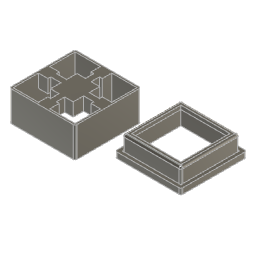
Eyebrow Warning Buttons v9 (Autodesk Fusion 360 design; units mm, degrees)
Autodesk Fusion 360 part; units mm, degrees
sketch "Sketch1" plane through (0, 0, 0) normal (0, 0, 1) x (1, 0, 0)
  line L0 (2.45, 3) -> (-2.45, 3)
  line L1 (-2.45, 3) -> (-2.45, -3)
  line L2 (-2.45, -3) -> (2.45, -3)
  line L3 (2.45, -3) -> (2.45, 3)
  line L4 (2.45, 3) -> (-2.45, -3) construction
  line L5 (-2.45, 3) -> (2.45, -3) construction
  line L6 (8.7, 8.7) -> (-8.7, 8.7)
  line L7 (-8.7, 8.7) -> (-8.7, -8.7)
  line L8 (-8.7, -8.7) -> (8.7, -8.7)
  line L9 (8.7, -8.7) -> (8.7, 8.7)
  line L10 (8.7, 8.7) -> (-8.7, -8.7) construction
  line L11 (-8.7, 8.7) -> (8.7, -8.7) construction
  line L12 (-8.7, 1.5) -> (-5.7, 1.5)
  line L13 (-5.7, 1.5) -> (-5.7, -1.5)
  line L14 (-5.7, -1.5) -> (-8.7, -1.5)
  line L15 (-8.7, -1.5) -> (-8.7, 1.5)
  line L16 (-1.5, 8.7) -> (1.5, 8.7)
  line L17 (1.5, 8.7) -> (1.5, 5.7)
  line L18 (1.5, 5.7) -> (-1.5, 5.7)
  line L19 (-1.5, 5.7) -> (-1.5, 8.7)
  line L20 (-1.5, -8.7) -> (1.5, -8.7)
  line L21 (1.5, -8.7) -> (1.5, -5.7)
  line L22 (1.5, -5.7) -> (-1.5, -5.7)
  line L23 (-1.5, -5.7) -> (-1.5, -8.7)
  line L24 (8.7, 1.5) -> (5.7, 1.5)
  line L25 (5.7, 1.5) -> (5.7, -1.5)
  line L26 (5.7, -1.5) -> (8.7, -1.5)
  line L27 (8.7, -1.5) -> (8.7, 1.5)
  line L28 (-8.2, 8.2) -> (8.2, 8.2)
  line L29 (8.2, 8.2) -> (8.2, -8.2)
  line L30 (8.2, -8.2) -> (-8.2, -8.2)
  line L31 (-8.2, -8.2) -> (-8.2, 8.2)
  line L32 (-8.2, 8.2) -> (8.2, -8.2) construction
  line L33 (8.2, 8.2) -> (-8.2, -8.2) construction
  line L34 (-3, 3.5) -> (3, 3.5)
  line L35 (3, 3.5) -> (3, -3.5)
  line L36 (3, -3.5) -> (-3, -3.5)
  line L37 (-3, -3.5) -> (-3, 3.5)
  line L38 (-3, 3.5) -> (3, -3.5) construction
  line L39 (3, 3.5) -> (-3, -3.5) construction
  line L40 (-6.05, 0.75) -> (-2.8, 0.75)
  line L41 (-2.8, 0.75) -> (-2.8, -0.75)
  line L42 (-2.8, -0.75) -> (-6.05, -0.75)
  line L43 (-6.05, -0.75) -> (-6.05, 0.75)
  line L44 (-0.75, -6.05) -> (0.75, -6.05)
  line L45 (0.75, -6.05) -> (0.75, -3.5)
  line L46 (0.75, -3.5) -> (-0.75, -3.5)
  line L47 (-0.75, -3.5) -> (-0.75, -6.05)
  line L48 (6.05, -0.75) -> (3, -0.75)
  line L49 (3, -0.75) -> (3, 0.75)
  line L50 (3, 0.75) -> (6.05, 0.75)
  line L51 (6.05, 0.75) -> (6.05, -0.75)
  line L52 (-0.75, 6.05) -> (0.75, 6.05)
  line L53 (0.75, 6.05) -> (0.75, 3.5)
  line L54 (0.75, 3.5) -> (-0.75, 3.5)
  line L55 (-0.75, 3.5) -> (-0.75, 6.05)
  point P0 (8.7, 0)
  point P1 (0, 8.7)
  point P2 (0, -8.7)
  point P3 (-5.7, 0)
  point P4 (0, -5.7)
  point P5 (5.7, 0)
  point P6 (0, 5.7)
  dimension "d1" = 4.9
  dimension "d2" = 6
  dimension "d3" = 17.4
  dimension "d4" = 17.4
  dimension "d7" = 3
  dimension "d8" = 3
  dimension "d15" = 3
  dimension "d16" = 3
  dimension "d17" = 3
  dimension "d18" = 3
  dimension "d19" = 3
  dimension "d20" = 3
  dimension "d21" = 16.4
  dimension "d22" = 16.4
  dimension "d23" = 6
  dimension "d24" = 7
  dimension "d31" = 1.5
  constraint horizontal L0
  constraint perpendicular L0 L1
  constraint parallel L0 L2
  constraint parallel L1 L3
  constraint coincident L4 origin
  constraint coincident L5 origin
  constraint horizontal L6
  constraint perpendicular L6 L7
  constraint parallel L6 L8
  constraint parallel L7 L9
  constraint coincident L10 origin
  constraint coincident L11 origin
  constraint horizontal L12
  constraint vertical L13
  constraint horizontal L14
  constraint vertical L15
  constraint midpoint L9 P0
  constraint midpoint L6 P1
  constraint midpoint L8 P2
  constraint horizontal L16
  constraint vertical L17
  constraint horizontal L18
  constraint vertical L19
  constraint horizontal L20
  constraint vertical L21
  constraint horizontal L22
  constraint vertical L23
  constraint horizontal L24
  constraint vertical L25
  constraint horizontal L26
  constraint vertical L27
  constraint horizontal L28
  constraint perpendicular L28 L29
  constraint parallel L28 L30
  constraint parallel L29 L31
  constraint coincident L32 origin
  constraint coincident L33 origin
  constraint horizontal L34
  constraint perpendicular L34 L35
  constraint parallel L34 L36
  constraint parallel L35 L37
  constraint coincident L38 origin
  constraint coincident L39 origin
  constraint midpoint L13 P3
  constraint horizontal L40
  constraint vertical L41
  constraint horizontal L42
  constraint vertical L43
  constraint midpoint L22 P4
  constraint horizontal L44
  constraint vertical L45
  constraint horizontal L46
  constraint vertical L47
  constraint coincident L36 L45.end
  constraint midpoint L25 P5
  constraint horizontal L48
  constraint vertical L49
  constraint horizontal L50
  constraint vertical L51
  constraint coincident L35 L49.end
  constraint midpoint L18 P6
  constraint horizontal L52
  constraint vertical L53
  constraint horizontal L54
  constraint vertical L55
  constraint coincident L34 L53.end
  measures "d1" distance of L1.end L2.end
  measures "d2" distance of L0.end L1.end
  measures "d3" distance of L7.end L8.end
  measures "d4" distance of L6.end L7.end
  measures "d7" distance of L12.start L12.end
  measures "d8" distance of L12.start L14.end
  measures "d15" distance of L16.start L16.end
  measures "d16" distance of L16.start L18.end
  measures "d17" distance of L20.start L20.end
  measures "d18" distance of L20.start L22.end
  measures "d19" distance of L24.start L24.end
  measures "d20" distance of L24.start L26.end
  measures "d21" distance of L29.end L30.end
  measures "d22" distance of L28.end L29.end
  measures "d23" distance of L35.end L36.end
  measures "d24" distance of L34.end L35.end
  measures "d31" distance of L40.start L42.end
extrude "Extrude1" add sketch "Sketch1" against normal blind 6.5 contours L6 L9 L17 L24 L28 L29 | L6 L16 L17 L19 L28 | L9 L24 L26 L27 L29 | L6 L7 L12 L19 L28 L31 | L17 L18 L19 L28 L52 L53 L55 | L8 L9 L21 L26 L29 L30 | L24 L25 L26 L29 L48 L50 L51 | L7 L12 L14 L15 L31 | L18 L52 L53 L55 | L8 L20 L21 L23 L30 | L25 L48 L50 L51 | L7 L8 L14 L23 L30 L31 | L12 L13 L14 L31 L40 L42 L43 | L21 L22 L23 L30 L44 L45 L47 | L13 L40 L42 L43 | L22 L44 L45 L47 makes body 1
fillet "Fillet1" radius 0.5 4 edges at (-8.7, 8.7, -3.25) (-8.7, -8.7, -3.25) (8.7, -8.7, -3.25) (8.7, 8.7, -3.25) on bodies 1
extrude "Extrude2" add sketch "Sketch1" against normal blind 2 separate body contours L18 L34 L53 L54 L55 | L25 L35 L48 L49 L50 | L34 L35 L36 L37 L40 L41 L42 L46 L49 L54 | L13 L37 L40 L42 | L22 L36 L45 L46 L47 | L37 L40 L41 L42 makes body 2
extrude "Extrude3" add sketch "Sketch1" along normal blind 1.5 contours L0 L1 L2 L3 | L6 L9 L17 L24 L28 L29 | L6 L16 L17 L19 L28 | L9 L24 L26 L27 L29 | L6 L7 L12 L19 L28 L31 | L17 L18 L19 L28 L52 L53 L55 | L8 L9 L21 L26 L29 L30 | L24 L25 L26 L29 L48 L50 L51 | L7 L12 L14 L15 L31 | L18 L34 L53 L54 L55 | L18 L52 L53 L55 | L8 L20 L21 L23 L30 | L25 L48 L50 L51 | L25 L35 L48 L49 L50 | L7 L8 L14 L23 L30 L31 | L12 L13 L14 L31 L40 L42 L43 | L34 L35 L36 L37 L40 L41 L42 L46 L49 L54 | L21 L22 L23 L30 L44 L45 L47 | L13 L37 L40 L42 | L13 L40 L42 L43 | L22 L44 L45 L47 | L22 L36 L45 L46 L47 | L37 L40 L41 L42 bodies 1 2
fillet "Fillet2" radius 0.5 4 edges at (-8.7, 8.7, 0.75) (8.7, 8.7, 0.75) (-8.7, -8.7, 0.75) (8.7, -8.7, 0.75) on bodies 1
sketch "Sketch2" plane through (0, 0, 0) normal (0, 0, 1) x (1, 0, 0)
  line L0 (34.75, 8.75) -> (19.25, 8.75)
  line L1 (19.25, 8.75) -> (19.25, -6.75)
  line L2 (19.25, -6.75) -> (34.75, -6.75)
  line L3 (34.75, -6.75) -> (34.75, 8.75)
  line L4 (34.75, 8.75) -> (19.25, -6.75) construction
  line L5 (19.25, 8.75) -> (34.75, -6.75) construction
  line L6 (33.5, 7.5) -> (20.5, 7.5)
  line L7 (20.5, 7.5) -> (20.5, -5.5)
  line L8 (20.5, -5.5) -> (33.5, -5.5)
  line L9 (33.5, -5.5) -> (33.5, 7.5)
  line L10 (33.5, 7.5) -> (20.5, -5.5) construction
  line L11 (20.5, 7.5) -> (33.5, -5.5) construction
  line L12 (35.7, 9.7) -> (18.3, 9.7)
  line L13 (18.3, 9.7) -> (18.3, -7.7)
  line L14 (18.3, -7.7) -> (35.7, -7.7)
  line L15 (35.7, -7.7) -> (35.7, 9.7)
  line L16 (35.7, 9.7) -> (18.3, -7.7) construction
  line L17 (18.3, 9.7) -> (35.7, -7.7) construction
  line L18 (34.25, 8.25) -> (19.75, 8.25)
  line L19 (19.75, 8.25) -> (19.75, -6.25)
  line L20 (19.75, -6.25) -> (34.25, -6.25)
  line L21 (34.25, -6.25) -> (34.25, 8.25)
  line L22 (34.25, 8.25) -> (19.75, -6.25) construction
  line L23 (19.75, 8.25) -> (34.25, -6.25) construction
  point P0 (27, 1)
  point P1 (27, 1)
  point P2 (27, 1)
  point P3 (27, 1)
  dimension "d38" = 15.5
  dimension "d39" = 15.5
  dimension "d40" = 13
  dimension "d41" = 13
  dimension "d46" = 17.4
  dimension "d47" = 17.4
  dimension "d50" = 14.5
  dimension "d51" = 14.5
  constraint horizontal L0
  constraint perpendicular L0 L1
  constraint parallel L0 L2
  constraint parallel L1 L3
  constraint coincident L4 P3
  constraint coincident L5 P3
  constraint horizontal L6
  constraint perpendicular L6 L7
  constraint parallel L6 L8
  constraint parallel L7 L9
  constraint coincident L10 P3
  constraint coincident L11 P3
  constraint coincident P3 P2
  constraint horizontal L12
  constraint perpendicular L12 L13
  constraint parallel L12 L14
  constraint parallel L13 L15
  constraint coincident L16 P3
  constraint coincident L17 P3
  constraint horizontal L18
  constraint perpendicular L18 L19
  constraint parallel L18 L20
  constraint parallel L19 L21
  constraint coincident L22 P3
  constraint coincident L23 P3
  measures "d38" distance of L1.end L2.end
  measures "d39" distance of L0.end L1.end
  measures "d40" distance of L7.end L8.end
  measures "d41" distance of L6.end L7.end
  measures "d46" distance of L13.end L14.end
  measures "d47" distance of L12.end L13.end
  measures "d50" distance of L19.end L20.end
  measures "d51" distance of L18.end L19.end
extrude "Extrude4" add sketch "Sketch2" along normal blind 4 separate body contours L0 L1 L2 L3 | L18 L19 L20 L21 makes body 3
fillet "Fillet3" radius 0.5 4 edges at (34.75, -6.75, 2) (34.75, 8.75, 2) (19.25, 8.75, 2) (19.25, -6.75, 2) on bodies 3
fillet "Fillet4" radius 0.6 8 edges at (34.6036, 8.6036, 4) (27, 8.75, 4) (19.3964, 8.6036, 4) (19.25, 1, 4) (19.3964, -6.6036, 4) (27, -6.75, 4) (34.6036, -6.6036, 4) (34.75, 1, 4) on bodies 3
extrude "Extrude5" add sketch "Sketch2" against normal blind 1.5 separate body contours L12 L13 L14 L15 makes body 4
extrude "Extrude6" cut sketch "Sketch2" along normal blind 3 contours L18 L19 L20 L21 bodies 3
extrude "Extrude7" add 1 faces at (34.5833, -1.4167, 0) along direction (0, 0, -1) blind 1.5 on bodies 3 bodies 3 4
fillet "Fillet5" radius 0.5 4 edges at (35.7, -7.7, -0.75) (35.7, 9.7, -0.75) (18.3, -7.7, -0.75) (18.3, 9.7, -0.75) on bodies 3
sketch "Sketch3" plane through (0, 0, -6.5) normal (0, 0, -1) x (1, 0, 0)
  arc A0 (8.2, -8.7) -> (8.7, -8.2) centre (8.2, -8.2) ccw
  line L0 (8.7, -8.2) -> (8.7, 8.2)
  arc A1 (8.7, 8.2) -> (8.2, 8.7) centre (8.2, 8.2) ccw
  line L1 (8.2, 8.7) -> (-8.2, 8.7)
  arc A2 (-8.2, 8.7) -> (-8.7, 8.2) centre (-8.2, 8.2) ccw
  line L2 (-8.7, 8.2) -> (-8.7, -8.2)
  arc A3 (-8.7, -8.2) -> (-8.2, -8.7) centre (-8.2, -8.2) ccw
  line L3 (-8.2, -8.7) -> (8.2, -8.7)
  line L4 (1.5, -8.2) -> (1.5, -5.7)
  line L5 (1.5, -5.7) -> (-1.5, -5.7)
  line L6 (-1.5, -5.7) -> (-1.5, -8.2)
  line L7 (-1.5, -8.2) -> (-8.2, -8.2)
  line L8 (-8.2, -8.2) -> (-8.2, -1.5)
  line L9 (-8.2, -1.5) -> (-5.7, -1.5)
  line L10 (-5.7, -1.5) -> (-5.7, 1.5)
  line L11 (-5.7, 1.5) -> (-8.2, 1.5)
  line L12 (-8.2, 1.5) -> (-8.2, 8.2)
  line L13 (-8.2, 8.2) -> (-1.5, 8.2)
  line L14 (-1.5, 8.2) -> (-1.5, 5.7)
  line L15 (-1.5, 5.7) -> (1.5, 5.7)
  line L16 (1.5, 5.7) -> (1.5, 8.2)
  line L17 (1.5, 8.2) -> (8.2, 8.2)
  line L18 (8.2, 8.2) -> (8.2, 1.5)
  line L19 (8.2, 1.5) -> (5.7, 1.5)
  line L20 (5.7, 1.5) -> (5.7, -1.5)
  line L21 (5.7, -1.5) -> (8.2, -1.5)
  line L22 (8.2, -1.5) -> (8.2, -8.2)
  line L23 (8.2, -8.2) -> (1.5, -8.2)
  line L24 (5.7, -1.5) -> (8.2, -1.5)
  line L25 (8.2, -1.5) -> (8.2, 1.5)
  line L26 (8.2, 1.5) -> (5.7, 1.5)
  line L27 (5.7, 1.5) -> (5.7, -1.5)
  line L28 (-5.7, -1.5) -> (-8.2, -1.5)
  line L29 (-8.2, -1.5) -> (-8.2, 1.5)
  line L30 (-8.2, 1.5) -> (-5.7, 1.5)
  line L31 (-5.7, 1.5) -> (-5.7, -1.5)
  constraint horizontal L24
  constraint vertical L25
  constraint horizontal L26
  constraint vertical L27
  constraint coincident L18.end L19.start
  constraint coincident L20.end L21.start
  constraint horizontal L28
  constraint vertical L29
  constraint horizontal L30
  constraint vertical L31
  constraint coincident L11.end L12.start
  constraint coincident L9.end L10.start
extrude "Extrude8" cut sketch "Sketch3" against normal blind 4.5 contours L19 L20 L21 L24 L25 L26 L27 | L9 L10 L11 L28 L29 L30 L31 bodies 1
